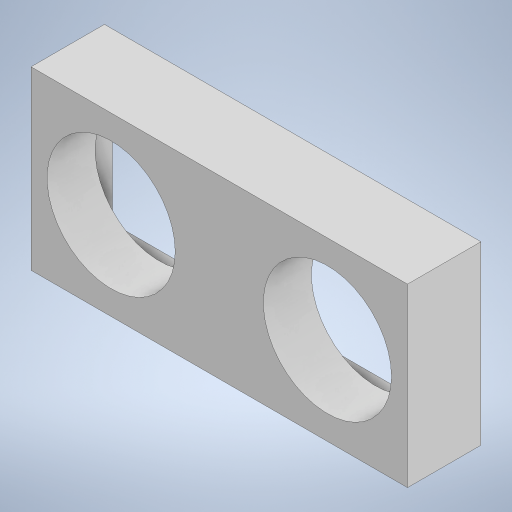
# Autodesk Inventor part: Sonar
Saved by Autodesk Inventor 2024.1 (Build 281209000, 209)
## iProperties
Created: 2024-05-13
Part Number: Sonar
Material: Generic
Document SubType Name: Modeling
Designer: cyan924
Density: 1 g/cm^3
Appearance: Default
Author: cyan924
Autodesk Inventor part; units mm, degrees
ref_plane "YZ Plane" through (0, 0, 0) normal (1, 0, 0) x (0, 1, 0)
ref_plane "XZ Plane" through (0, 0, 0) normal (0, 1, 0) x (-1, 0, 0)
ref_plane "XY Plane" through (0, 0, 0) normal (0, 0, 1) x (1, 0, 0)
sketch "Sketch1" plane through (0, 0, 0) normal (0, 0, 1) x (1, 0, 0)
  line L0 (0, 0) -> (45, 0) construction
  line L1 (45, 0) -> (45, 20) construction
  line L2 (45, 20) -> (0, 20) construction
  line L3 (0, 20) -> (0, 0) construction
  line L4 (0, 0) -> (9, 0) construction
  line L5 (9, 0) -> (9, 10) construction
  line L6 (45, 0) -> (36, 0) construction
  line L7 (36, 0) -> (36, 10) construction
  circle A0 centre (36, 10) radius 8
  circle A1 centre (9, 10) radius 8
  line L8 (45, 0) -> (46, 0) construction
  line L9 (46, 0) -> (46, -1) construction
  line L10 (0, 20) -> (-1, 20) construction
  line L11 (-1, 20) -> (-1, 21) construction
  line L12 (-1, 21) -> (46, 21)
  line L13 (46, 21) -> (46, -1)
  line L14 (46, -1) -> (-1, -1)
  line L15 (-1, -1) -> (-1, 21)
  line L16 (45, 0) -> (0, 0)
  line L17 (0, 0) -> (0, 20)
  line L18 (0, 20) -> (45, 20)
  line L19 (45, 20) -> (45, 0)
  dimension "d2" = 45
  dimension "d3" = 20
  dimension "d4" = 9
  dimension "d5" = 10
  dimension "d6" = 9
  dimension "d7" = 10
  dimension "d8" = 16
  dimension "d9" = 16
  dimension "d10" = 1
  dimension "d11" = 1
  dimension "d12" = 1
  dimension "d13" = 1
  constraints: 40 end point, 7 perpendicular, 6 parallel, 5 horizontal, 2 centre point, 2 coincident, 2 point on line
  measures "d2" distance of L2.end L1.end
  measures "d3" distance of L1.end L0.end
  measures "d4" distance of L0.start L4.end
  measures "d5" distance of L4.end L5.end
  measures "d6" distance of L0.end L6.end
  measures "d7" distance of L6.end L7.end
  measures "d8" diameter of A0
  measures "d9" diameter of A1
  measures "d10" distance of L0.end L8.end
  measures "d11" distance of L8.end L9.end
  measures "d12" distance of L2.end L10.end
  measures "d13" distance of L10.end L11.end
extrude "Extrusion1" add sketch "Sketch1" along normal blind 9.169 contours L12 L13 L14 L15 | L16 L17 L18 L19
sketch "Sketch2" plane through (0, 0, 0) normal (0, 0, -1) x (-1, 0, 0)
  line L0 (0, 0) -> (-45, 0)
  line L1 (-45, 0) -> (-45, 20)
  line L2 (-45, 20) -> (0, 20)
  line L3 (0, 20) -> (0, 0)
  dimension "d14" = 45
  dimension "d15" = 20
  constraints: 8 end point, 2 parallel, 1 horizontal, 1 perpendicular
  measures "d14" distance of L1.end L2.end
  measures "d15" distance of L0.end L1.end
extrude "Extrusion2" cut sketch "Sketch2" against normal blind 3.169
equation "\"d2\" = wsonar"
equation "\"d3\" = hsonar"
equation "\"d10\" = thickness"
equation "\"d11\" = thickness"
equation "\"d12\" = thickness"
equation "\"d13\" = thickness"
equation "\"d14\" = wsonar"
equation "\"d15\" = hsonar"
equation "\"wsonar\" = 45"
equation "\"hsonar\" = 20"
equation "\"thickness\" = 1"
body "Solid1"
